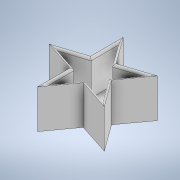
# Autodesk Inventor part: StarP
Saved by Autodesk Inventor 2020.3 (Build 243373000, 373)
## iProperties
Created: 2021-05-21
Part Number: StarP
Material: Generic
Document SubType Name: Modeling
Designer: patry
Density: 1 g/cm^3
Appearance: Default
Author: patry
Autodesk Inventor part; units mm, degrees
ref_plane "YZ Plane" through (0, 0, 0) normal (1, 0, 0) x (0, 1, 0)
ref_plane "XZ Plane" through (0, 0, 0) normal (0, 1, 0) x (-1, 0, 0)
ref_plane "XY Plane" through (0, 0, 0) normal (0, 0, 1) x (1, 0, 0)
sketch "Sketch1" plane through (0, 0, 0) normal (0, 1, 0) x (-1, 0, 0)
  circle A0 centre (0, 0) radius 52.5
  line L0 (52.5, 0) -> (16.2234, -49.9305)
  line L1 (16.2234, -49.9305) -> (-42.4734, -30.8587)
  line L2 (-42.4734, -30.8587) -> (-42.4734, 30.8587)
  line L3 (-42.4734, 30.8587) -> (16.2234, 49.9305)
  line L4 (16.2234, 49.9305) -> (52.5, 0)
  line L5 (52.5, 0) -> (-42.4734, 30.8587)
  line L6 (-42.4734, -30.8587) -> (52.5, 0)
  line L7 (16.2234, -49.9305) -> (16.2234, 49.9305)
  line L8 (-42.4734, -30.8587) -> (16.2234, 49.9305)
  line L9 (-42.4734, 30.8587) -> (16.2234, -49.9305)
  point P0 (16.2234, -11.787)
  point P1 (16.2234, 11.787)
  point P2 (-6.1968, 19.0717)
  point P3 (-20.0532, 0)
  point P4 (-6.1968, -19.0717)
  constraints: 20 end point, 2 coincident, 1 horizontal alignment, 1 vertical, 13 other
extrude "Extrusion1" add sketch "Sketch1" along normal blind 5 contours L6 L7 L5 | L7 L5 L8 | L9 L6 L7 | L7 L6 L9 L8 L5 | L5 L8 L9 | L8 L9 L6
sketch "Sketch2" plane through (0, 5, 0) normal (0, 1, 0) x (1, 0, 0)
  circle A0 centre (0, 0) radius 4.25
  dimension "d3" = 8.5
  constraints: 1 centre point, 1 coincident
  measures "d3" diameter of A0
extrude "Extrusion2" cut sketch "Sketch2" against normal blind 2
sketch "Sketch3" plane through (0, 3, 0) normal (0, 1, 0) x (1, 0, 0)
  circle A0 centre (0, 0) radius 2.5
  dimension "d6" = 5
  constraints: 1 centre point, 1 coincident
  measures "d6" diameter of A0
extrude "Extrusion3" cut sketch "Sketch3" against normal through all
sketch "Sketch4" plane through (0, 5, 0) normal (0, 1, 0) x (1, 0, 0)
  line L0 (-16.2234, 11.787) -> (-52.5, 0) projected
  line L1 (-52.5, 0) -> (-16.2234, 11.787)
  line L2 (6.1968, 19.0717) -> (-16.2234, 49.9305) projected
  line L3 (-16.2234, 11.787) -> (-16.2234, 49.9305)
  line L4 (-16.2234, 49.9305) -> (6.1968, 19.0717)
  line L5 (42.4734, 30.8587) -> (6.1968, 19.0717) projected
  line L6 (6.1968, 19.0717) -> (42.4734, 30.8587)
  line L7 (42.4734, 30.8587) -> (20.0532, 0)
  line L8 (20.0532, 0) -> (42.4734, -30.8587)
  line L9 (-16.2234, -49.9305) -> (6.1968, -19.0717) projected
  line L10 (42.4734, -30.8587) -> (6.1968, -19.0717)
  line L11 (6.1968, -19.0717) -> (-16.2234, -49.9305)
  line L12 (-16.2234, -11.787) -> (-16.2234, -49.9305) projected
  line L13 (-16.2234, -49.9305) -> (-16.2234, -11.787)
  line L14 (-16.2234, -11.787) -> (-52.5, 0)
  line L15 (-52.5, 0) -> (-16.2234, -11.787) projected
  line L16 (-16.2234, -49.9305) -> (-15.4508, -47.5528)
  line L17 (-52.5, 0) -> (-44.4, 0)
  line L18 (-44.4, 0) -> (-13.7204, 42.2269)
  line L19 (-13.7204, 42.2269) -> (35.9204, 26.0977)
  line L20 (35.9204, 26.0977) -> (35.9204, -26.0977)
  line L21 (35.9204, -26.0977) -> (-13.7204, -42.2269)
  line L22 (-13.7204, -42.2269) -> (-44.4, 0)
  line L23 (-44.4, 0) -> (-13.7204, -42.2269)
  line L24 (-13.7204, -42.2269) -> (-13.7204, 42.2269)
  line L25 (-16.2234, -11.787) -> (-16.2234, -49.9305) projected
  line L26 (-13.7204, 42.2269) -> (35.9204, -26.0977)
  line L27 (35.9204, -26.0977) -> (-44.4, 0)
  line L28 (-44.4, 0) -> (35.9204, 26.0977)
  line L29 (35.9204, 26.0977) -> (-13.7204, -42.2269)
  line L30 (-16.2234, -49.9305) -> (6.1968, -19.0717) projected
  point P0 (0, 0)
  point P1 (0, 0)
  point P2 (5.2407, 16.1292)
  point P3 (16.9593, 0)
  point P4 (5.2407, -16.1292)
  point P5 (-13.7204, -9.9684)
  point P6 (-13.7204, 9.9684)
  dimension "d10" = 2.5
  dimension "d11" = 8.1
  constraints: 46 end point, 8 collinear, 4 parallel, 1 coincident, 1 horizontal, 1 perpendicular, 1 vertical, 11 other
  measures "d10" distance of L9.start L16.end
  measures "d11" distance of L0.end L17.end
extrude "Extrusion4" add sketch "Sketch4" along normal blind 40 contours L3 L18 L24 L28 L0 | L18 L17 L0 | L3 L2 L19 L18 | L17 L22 L14 | L27 L24 L22 L12 L14 | L19 L2 L5 L28 L26 | L22 L21 L9 L12 | L29 L27 L21 L10 L9 | L5 L7 L20 L19 | L29 L20 L7 L8 L26 | L20 L8 L10 L21
fillet "Fillet1" radius 2.5 10 edges at (-13.7204, 45, 26.0977) (-29.0602, 45, 4.9842) (-29.0602, 45, -4.9842) (-13.7204, 45, -26.0977) (-4.2398, 45, -29.1781) (20.5805, 45, -21.1135) (26.4398, 45, -13.0488) (26.4398, 45, 13.0488) (20.5805, 45, 21.1135) (-4.2398, 45, 29.1781)
body "Solid1"
